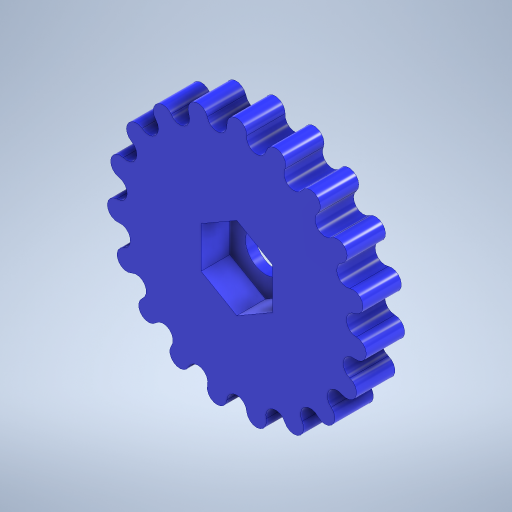
# Autodesk Inventor part: X_belt3
Saved by Autodesk Inventor 2023 (Build 270158000, 158)
## iProperties
Created: 2023-03-07
Part Number: X_belt3
Material: Типовые
Document SubType Name: Modeling
Designer: Josh
Density: 1 g/cm^3
Appearance: Синий — малярная краска — глянцевая
Author: Josh
Autodesk Inventor part; units mm, degrees
ref_plane "YZ Plane" through (0, 0, 0) normal (1, 0, 0) x (0, 1, 0)
ref_plane "XZ Plane" through (0, 0, 0) normal (0, 1, 0) x (-1, 0, 0)
ref_plane "XY Plane" through (0, 0, 0) normal (0, 0, 1) x (1, 0, 0)
sketch "Эскиз1" plane through (0, 0, 0) normal (0, 0, 1) x (1, 0, 0)
  line L0 (0, 4.3013) -> (3.725, 2.1506)
  line L1 (3.725, 2.1506) -> (3.725, -2.1506)
  line L2 (3.725, -2.1506) -> (0, -4.3013)
  line L3 (0, -4.3013) -> (-3.725, -2.1506)
  line L4 (-3.725, -2.1506) -> (-3.725, 2.1506)
  line L5 (-3.725, 2.1506) -> (0, 4.3013)
  circle A0 centre (0, 0) radius 12.5 construction
  arc A1 (1.0318, 12.4573) -> (-1.0292, 12.4147) centre (0, 12.5) ccw
  arc A2 (-1.0292, 12.4147) -> (-3.069, 12.1174) centre (-2.0583, 12.3294) ccw construction
  arc A3 (-3.069, 12.1174) -> (-1.0292, 12.4147) centre (-2.0583, 12.3294) ccw
  arc A4 (-1.0292, 12.4147) -> (1.0318, 12.4573) centre (0, 12.5) ccw construction
  arc A5 (-3.069, 12.1174) -> (-5.0044, 11.4079) centre (-4.0587, 11.8227) ccw
  arc A6 (-5.0044, 11.4079) -> (-6.8372, 10.4643) centre (-5.9501, 10.993) ccw construction
  arc A7 (-6.8372, 10.4643) -> (-5.0044, 11.4079) centre (-5.9501, 10.993) ccw
  arc A8 (-5.0044, 11.4079) -> (-3.069, 12.1174) centre (-4.0587, 11.8227) ccw construction
  arc A9 (-6.8372, 10.4643) -> (-8.4374, 9.1648) centre (-7.6777, 9.8643) ccw
  arc A10 (-8.4374, 9.1648) -> (-9.8645, 7.6773) centre (-9.1971, 8.4654) ccw construction
  arc A11 (-9.8645, 7.6773) -> (-8.4374, 9.1648) centre (-9.1971, 8.4654) ccw
  arc A12 (-8.4374, 9.1648) -> (-6.8372, 10.4643) centre (-7.6777, 9.8643) ccw construction
  arc A13 (-9.8645, 7.6773) -> (-10.9561, 5.9286) centre (-10.4646, 6.8369) ccw
  arc A14 (-10.9561, 5.9286) -> (-11.8229, 4.0583) centre (-11.4475, 5.0204) ccw construction
  arc A15 (-11.8229, 4.0583) -> (-10.9561, 5.9286) centre (-11.4475, 5.0204) ccw
  arc A16 (-10.9561, 5.9286) -> (-9.8645, 7.6773) centre (-10.4646, 6.8369) ccw construction
  arc A17 (-11.8229, 4.0583) -> (-12.2874, 2.05) centre (-12.1175, 3.0686) ccw
  arc A18 (-12.2874, 2.05) -> (-12.5, -0.0004) centre (-12.4574, 1.0314) ccw construction
  arc A19 (-12.5, -0.0004) -> (-12.2874, 2.05) centre (-12.4574, 1.0314) ccw
  arc A20 (-12.2874, 2.05) -> (-11.8229, 4.0583) centre (-12.1175, 3.0686) ccw construction
  arc A21 (-12.5, -0.0004) -> (-12.2873, -2.0508) centre (-12.4573, -1.0322) ccw
  arc A22 (-12.2873, -2.0508) -> (-11.8226, -4.0592) centre (-12.1173, -3.0694) ccw construction
  arc A23 (-11.8226, -4.0592) -> (-12.2873, -2.0508) centre (-12.1173, -3.0694) ccw
  arc A24 (-12.2873, -2.0508) -> (-12.5, -0.0004) centre (-12.4573, -1.0322) ccw construction
  arc A25 (-11.8226, -4.0592) -> (-10.9556, -5.9294) centre (-11.4472, -5.0212) ccw
  arc A26 (-10.9556, -5.9294) -> (-9.864, -7.678) centre (-10.4641, -6.8376) ccw construction
  arc A27 (-9.864, -7.678) -> (-10.9556, -5.9294) centre (-10.4641, -6.8376) ccw
  arc A28 (-10.9556, -5.9294) -> (-11.8226, -4.0592) centre (-11.4472, -5.0212) ccw construction
  arc A29 (-9.864, -7.678) -> (-8.4368, -9.1654) centre (-9.1965, -8.466) ccw
  arc A30 (-8.4368, -9.1654) -> (-6.8365, -10.4648) centre (-7.677, -9.8648) ccw construction
  arc A31 (-6.8365, -10.4648) -> (-8.4368, -9.1654) centre (-7.677, -9.8648) ccw
  arc A32 (-8.4368, -9.1654) -> (-9.864, -7.678) centre (-9.1965, -8.466) ccw construction
  arc A33 (-6.8365, -10.4648) -> (-5.0036, -11.4082) centre (-5.9493, -10.9934) ccw
  arc A34 (-5.0036, -11.4082) -> (-3.0681, -12.1176) centre (-4.0579, -11.823) ccw construction
  arc A35 (-3.0681, -12.1176) -> (-5.0036, -11.4082) centre (-4.0579, -11.823) ccw
  arc A36 (-5.0036, -11.4082) -> (-6.8365, -10.4648) centre (-5.9493, -10.9934) ccw construction
  arc A37 (-3.0681, -12.1176) -> (-1.0283, -12.4148) centre (-2.0574, -12.3295) ccw
  arc A38 (-1.0283, -12.4148) -> (1.0327, -12.4573) centre (0.0009, -12.5) ccw construction
  arc A39 (1.0327, -12.4573) -> (-1.0283, -12.4148) centre (0.0009, -12.5) ccw
  arc A40 (-1.0283, -12.4148) -> (-3.0681, -12.1176) centre (-2.0574, -12.3295) ccw construction
  arc A41 (1.0327, -12.4573) -> (3.0585, -12.076) centre (2.0574, -12.3295) ccw
  arc A42 (3.0585, -12.076) -> (5.0216, -11.447) centre (4.0596, -11.8224) ccw construction
  arc A43 (5.0216, -11.447) -> (3.0585, -12.076) centre (4.0596, -11.8224) ccw
  arc A44 (3.0585, -12.076) -> (1.0327, -12.4573) centre (2.0574, -12.3295) ccw construction
  arc A45 (5.0216, -11.447) -> (6.8138, -10.4286) centre (5.9493, -10.9934) ccw
  arc A46 (6.8138, -10.4286) -> (8.4663, -9.1962) centre (7.6784, -9.8637) ccw construction
  arc A47 (8.4663, -9.1962) -> (6.8138, -10.4286) centre (7.6784, -9.8637) ccw
  arc A48 (6.8138, -10.4286) -> (5.0216, -11.447) centre (5.9493, -10.9934) ccw construction
  arc A49 (8.4663, -9.1962) -> (9.8308, -7.6511) centre (9.1965, -8.466) ccw
  arc A50 (9.8308, -7.6511) -> (10.9936, -5.949) centre (10.4651, -6.8361) ccw construction
  arc A51 (10.9936, -5.949) -> (9.8308, -7.6511) centre (10.4651, -6.8361) ccw
  arc A52 (9.8308, -7.6511) -> (8.4663, -9.1962) centre (9.1965, -8.466) ccw construction
  arc A53 (10.9936, -5.949) -> (11.7824, -4.0445) centre (11.4472, -5.0212) ccw
  arc A54 (11.7824, -4.0445) -> (12.3296, -2.057) centre (12.1177, -3.0677) ccw construction
  arc A55 (12.3296, -2.057) -> (11.7824, -4.0445) centre (12.1177, -3.0677) ccw
  arc A56 (11.7824, -4.0445) -> (10.9936, -5.949) centre (11.4472, -5.0212) ccw construction
  arc A57 (12.3296, -2.057) -> (12.4573, 0.0004) centre (12.4573, -1.0322) ccw
  arc A58 (12.4573, 0.0004) -> (12.3294, 2.0579) centre (12.4572, 1.0331) ccw construction
  arc A59 (12.3294, 2.0579) -> (12.4573, 0.0004) centre (12.4572, 1.0331) ccw
  arc A60 (12.4573, 0.0004) -> (12.3296, -2.057) centre (12.4573, -1.0322) ccw construction
  arc A61 (12.3294, 2.0579) -> (11.7822, 4.0453) centre (12.1175, 3.0686) ccw
  arc A62 (11.7822, 4.0453) -> (10.9932, 5.9497) centre (11.4468, 5.022) ccw construction
  arc A63 (10.9932, 5.9497) -> (11.7822, 4.0453) centre (11.4468, 5.022) ccw
  arc A64 (11.7822, 4.0453) -> (12.3294, 2.0579) centre (12.1175, 3.0686) ccw construction
  arc A65 (10.9932, 5.9497) -> (9.8303, 7.6518) centre (10.4646, 6.8369) ccw
  arc A66 (9.8303, 7.6518) -> (8.4657, 9.1968) centre (9.1959, 8.4667) ccw construction
  arc A67 (8.4657, 9.1968) -> (9.8303, 7.6518) centre (9.1959, 8.4667) ccw
  arc A68 (9.8303, 7.6518) -> (10.9932, 5.9497) centre (10.4646, 6.8369) ccw construction
  arc A69 (8.4657, 9.1968) -> (6.8131, 10.429) centre (7.6777, 9.8643) ccw
  arc A70 (6.8131, 10.429) -> (5.0208, 11.4473) centre (5.9486, 10.9938) ccw construction
  arc A71 (5.0208, 11.4473) -> (6.8131, 10.429) centre (5.9486, 10.9938) ccw
  arc A72 (6.8131, 10.429) -> (8.4657, 9.1968) centre (7.6777, 9.8643) ccw construction
  arc A73 (5.0208, 11.4473) -> (3.0577, 12.0762) centre (4.0587, 11.8227) ccw
  arc A74 (3.0577, 12.0762) -> (1.0318, 12.4573) centre (2.0566, 12.3297) ccw construction
  arc A75 (1.0318, 12.4573) -> (3.0577, 12.0762) centre (2.0566, 12.3297) ccw
  arc A76 (3.0577, 12.0762) -> (5.0208, 11.4473) centre (4.0587, 11.8227) ccw construction
  circle A77 centre (0, 0) radius 2.1
  point P0 (-1.0318, 12.4573)
  point P1 (-5.0208, 11.4473)
  point P2 (-8.4657, 9.1968)
  point P3 (-10.9932, 5.9497)
  point P4 (-12.3294, 2.0579)
  point P5 (-12.3296, -2.057)
  point P6 (-10.9936, -5.949)
  point P7 (-8.4663, -9.1962)
  point P8 (-5.0216, -11.447)
  point P9 (-1.0327, -12.4573)
  point P10 (3.0681, -12.1176)
  point P11 (6.8365, -10.4648)
  point P12 (9.864, -7.678)
  point P13 (11.8226, -4.0592)
  point P14 (12.5, -0.0004)
  point P15 (11.8229, 4.0583)
  point P16 (9.8645, 7.6773)
  point P17 (6.8372, 10.4643)
  point P18 (3.069, 12.1174)
  point P19 (5.0208, 11.4473)
  point P20 (1.0318, 12.4573)
  point P21 (-3.069, 12.1174)
  point P22 (-9.8645, 7.6773)
  point P23 (-12.5, -0.0004)
  point P24 (-11.8226, -4.0592)
  point P25 (-9.864, -7.678)
  point P26 (-6.8365, -10.4648)
  point P27 (-3.0681, -12.1176)
  point P28 (1.0327, -12.4573)
  point P29 (5.0216, -11.447)
  point P30 (8.4663, -9.1962)
  point P31 (12.3296, -2.057)
  point P32 (12.3294, 2.0579)
  point P33 (10.9932, 5.9497)
  point P34 (8.4657, 9.1968)
  dimension "d0" = 7.45
  dimension "d1" = 25
  dimension "d6" = 360
  dimension "d8" = 4.2
  constraints: 176 point on circle, 78 centre point, 12 end point, 4 coincident, 2 equal radius, 2 vertical alignment, 204 other
  measures "d0" distance between parallel lines of L4 L1
  measures "d1" diameter of A0
  measures "d8" diameter of A77
extrude "Выдавливание1" add sketch "Эскиз1" along normal blind 4 contours A75 A73 A71 A69 A67 A65 A63 A61 A59 A57 A55 A53 A51 A49 A47 A45 A43 A41 A39 A37 A35 A33 A31 A29 A27 A25 A23 A21 A19 A17 A15 A13 A11 A9 A7 A5 A3 A1
extrude "Выдавливание2" add sketch "Эскиз1" along normal blind 1 contours L0 L1 L2 L3 L4 L5
